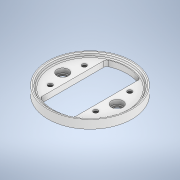
# Autodesk Inventor part: CarriageCap
Saved by Autodesk Inventor 2020 (Build 240168000, 168)
## iProperties
Created: 2019-07-20
Part Number: CarriageCap
Material: ABS Plastic
Document SubType Name: Modeling
Designer: Connor
Density: 1.06 g/cm^3
Appearance: White
Author: Connor
Autodesk Inventor part; units mm, degrees
ref_plane "YZ Plane" through (0, 0, 0) normal (1, 0, 0) x (0, 1, 0)
ref_plane "XZ Plane" through (0, 0, 0) normal (0, 1, 0) x (-1, 0, 0)
ref_plane "XY Plane" through (0, 0, 0) normal (0, 0, 1) x (1, 0, 0)
sketch "Sketch1" plane through (0, 0, 0) normal (0, 0, 1) x (1, 0, 0)
  line L0 (0, 0) -> (46.99, 0)
  line L1 (46.99, 0) -> (46.99, 9.525)
  line L2 (46.99, 9.525) -> (44.8564, 9.525)
  line L3 (44.8564, 9.525) -> (43.0233, 6.35)
  line L4 (43.0233, 6.35) -> (0, 6.35)
  line L5 (0, 6.35) -> (0, 0)
  dimension "d0" = 44.8564
  dimension "d2" = 9.525
  dimension "d3" = 60
  dimension "d4" = 46.99
  dimension "d7" = 3.175
  constraints: 12 end point, 3 perpendicular, 1 horizontal, 1 parallel
  measures "d0" distance from line of L2.end L5
  measures "d2" distance of L0.end L1.end
  measures "d3" angle of L4 L3
  measures "d4" distance between parallel lines of L5 L1
  measures "d7" distance between parallel lines of L2 L4
revolve "Revolution1" add sketch "Sketch1" angle 360 about axis through (0, 6.35, 0) along (0, -1, 0)
fillet "Fillet1" radius 1.5875 2 edges at (-44.8564, 9.525, 0) (-43.0233, 6.35, 0)
sketch "Sketch2" plane through (0, 6.35, 0) normal (0, 1, 0) x (1, 0, 0)
  circle A0 centre (0, 0) radius 41.275
  line L0 (-19.05, 36.6159) -> (-19.05, -36.6159)
  line L1 (19.05, -36.6159) -> (19.05, 36.6159)
  dimension "d8" = 82.55
  dimension "d9" = 38.1
  constraints: 4 end point, 4 point on circle, 2 vertical, 1 centre point, 1 coincident, 1 parallel
  measures "d8" diameter of A0
  measures "d9" distance between parallel lines of L1 L0
extrude "Extrusion1" cut sketch "Sketch2" against normal through all contours L1 A0 L0
sketch "Sketch3" plane through (0, 6.35, 0) normal (0, 1, 0) x (1, 0, 0)
  line L0 (0, 0) -> (-30.48, 0) construction
  line L1 (0, 0) -> (30.48, 0) construction
  dimension "d12" = 60.96
  constraints: 4 end point, 2 horizontal, 1 collinear
  measures "d12" distance of L1.end L0.end
hole "Hole1" at (-30.48, 6.35, 0) at (30.48, 6.35, 0) direction (0, -1, 0) diameter 8.89 end through all counterbore diameter 12.954 counterbore depth 4.7752
sketch "Sketch4" plane through (0, 0, 0) normal (0, -1, 0) x (1, 0, 0)
  line L0 (25.4, -19.05) -> (-25.4, -19.05) construction
  line L1 (-25.4, -19.05) -> (-25.4, 19.05) construction
  line L2 (-25.4, 19.05) -> (25.4, 19.05) construction
  line L3 (25.4, 19.05) -> (25.4, -19.05) construction
  line L4 (25.4, -19.05) -> (-25.4, 19.05) construction
  line L5 (25.4, 19.05) -> (-25.4, -19.05) construction
  point P0 (0, 0)
  point P1 (0, 0)
  dimension "d20" = 50.8
  dimension "d21" = 38.1
  constraints: 12 end point, 2 parallel, 1 coincident, 1 horizontal, 1 midpoint, 1 perpendicular
  measures "d20" distance of L0.start L0.end
  measures "d21" distance of L0.end L1.end
hole "Hole2" at (25.4, 0, -19.05) at (-25.4, 0, -19.05) at (-25.4, 0, 19.05) at (25.4, 0, 19.05) direction (0, 1, 0) diameter 5.207 end through all counterbore diameter 8.7313 counterbore depth 4.826
fillet "Fillet2" radius 3.175 4 edges at (19.05, 3.175, -36.6159) (19.05, 3.175, 36.6159) (-19.05, 3.175, 36.6159) (-19.05, 3.175, -36.6159)
body "Solid1"
